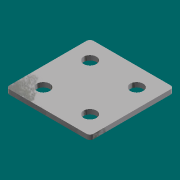
# Autodesk Inventor part: SHPTSD5-1
Saved by Autodesk Inventor 2016 (Build 200138000, 138)
## iProperties
Category: PARTsolutions
Company: MISUMI
Created: 2016-02-10
Part Number: SHPTSD5-1
Catalog Web Link: www.cadenas.de
Description: HPTSS, SHPTSS, HPTSSL, SHPTSSL, HPTSD, SHPTSD-1-Sheet Metal-1
Vendor: MISUMI
Document SubType Name: Modeling
Designer: psAdmin
Manufacturer: MISUMI
Mass: 19.1846 g
Surface Area: 28.1915 cm^2
Volume: 2.39807 cm^3
Density: 8 g/cm^3
Material: Stainless Steel
Appearance: Semi-Polished
PSOL_IDENT_0: {$CADENAS_DATA\23d-libs\misumi\metric\38_al_extrusions_blackets\hptss.prj},214 {VTYP=3D},{NB=SHPTSD5
PSOL_IDENT_1: -1},{LINA=SHPTSD5-1},{NN=HPTSS, SHPTSS, HPTSSL, SHPTSSL, HPTSD, SHPTSD-1},{DATE=17.07.2015 10:48:17}
PSOL_IDENT_2: ,{GEOMDATE=27.12.2010 00:00:00},{VERSION=},{LINEID=270},{LINESUBID=-1},{WBVAR=MAT,SHP,ALT1}  {NB=SHP
PSOL_IDENT_3: TSD5-1},{LINA=SHPTSD5-1},{KT=5},{PN=SHPTSD5-1},{TYPE=SHPTSD},{NO=5},{MAT=S},{MATALG= '','Low Carbon
PSOL_IDENT_4: Steel','S','304 Stainless Steel' },{ST=-},{SHP=SD},{ALT1=},{MASS=21},{A=36},{B=0},{T=2.0},{N=5.500},
PSOL_IDENT_5: {W=20.000},{R=1.500},{AB=SCB5-8},{NOB=4},{AN=HNTTSN5-8},{NON=4},{MASS1=11.000},{MASS2=22.000},{MASS3=
PSOL_IDENT_6: 21.000},{A1=18.000},{A2=36.000},{T1=2.300},{T2=2.000},{B1=36.000},{B2=80.000},{AB1=5-8},{AN1=5.000},
PSOL_IDENT_7: {SHPALG='SS', 'SHPTSS (Rectangular, 2 Holes)', 'SSL', 'SHPTSSL (Rectangular, 4 Holes)', 'SD'  , 'SHP
PSOL_IDENT_8: TSD (Square, 4 Holes)'},{M=5},{L=8.000},{NO1=5.000},{L1=8},{MAT1=1010 Steel (or Equivalent)},{MAT2=3
PSOL_IDENT_9: 16 Stainless Steel (or Equivalent)},{TT=1.200}
NN: HPTSS, SHPTSS, HPTSSL, SHPTSSL, HPTSD, SHPTSD-1
NT: Sheet Metal-1
NB: SHPTSD5-1
NBSYN: $PN.
LINA: SHPTSD5-1
PN: SHPTSD5-1
NO: 5
MAT: 304 Stainless Steel
ST: -
SHP: SHPTSD (Square, 4 Holes)
ALT1: w/o Fixing Bolt & Nut Set
MASS: 21
A: 36
B: 0
T: 2.0
N: 5.500
W: 20.000
R: 1.500
AB: SCB5-8
NOB: 4
AN: HNTTSN5-8
NON: 4
M: 5
L: 8.000
NO1: 5.000
L1: 8
MAT1: 1010 Steel (or Equivalent)
MAT2: 316 Stainless Steel (or Equivalent)
TT: 1.200
SUPPLIER: MISUMI
ARTICLENO: SHPTSD5-1
BOMINFO: SHPTSD5-1
CREATOR: CADENAS GmbH
Title: SHPTSD5-1
Author: Cadenas PARTsolutions
Comments: Sheet Metal-1
Autodesk Inventor part; units mm, degrees
sketch "Sketch_1" plane through (0, 0, 0) normal (0, 0, 1) x (1, 0, 0)
  arc A0 (-18, 1.5) -> (-16.5, 0) centre (-16.5, 1.5) ccw
  line L0 (-16.5, 0) -> (16.5, 0)
  arc A1 (16.5, 0) -> (18, 1.5) centre (16.5, 1.5) ccw
  line L1 (18, 1.5) -> (18, 34.5)
  arc A2 (18, 34.5) -> (16.5, 36) centre (16.5, 34.5) ccw
  line L2 (16.5, 36) -> (-16.5, 36)
  arc A3 (-16.5, 36) -> (-18, 34.5) centre (-16.5, 34.5) ccw
  line L3 (-18, 34.5) -> (-18, 1.5)
  circle A4 centre (10, 28) radius 2.75
  circle A5 centre (10, 8) radius 2.75
  circle A6 centre (-10, 28) radius 2.75
  circle A7 centre (-10, 8) radius 2.75
  constraints: 8 centre point, 8 end point, 8 point on circle
extrude "Extrusion1" add sketch "Sketch_1" against normal blind 2
ref_plane "to_bolt1_XY" through (-10, 8, 0) normal (0, 0, 1) x (1, 0, 0)
ref_plane "to_bolt1_YZ" through (-10, 8, 0) normal (1, 0, 0) x (0, 1, 0)
ref_plane "to_bolt1_ZX" through (-10, 8, 0) normal (0, 1, 0) x (0, 0, 1)
ref_plane "to_bolt2_XY" through (-10, 28, 0) normal (0, 0, 1) x (1, 0, 0)
ref_plane "to_bolt2_YZ" through (-10, 28, 0) normal (1, 0, 0) x (0, 1, 0)
ref_plane "to_bolt2_ZX" through (-10, 28, 0) normal (0, 1, 0) x (0, 0, 1)
ref_plane "to_dummy_XY" through (0, 18, 0) normal (0, 0, 1) x (1, 0, 0)
ref_plane "to_dummy_YZ" through (0, 18, 0) normal (1, 0, 0) x (0, 1, 0)
ref_plane "to_dummy_ZX" through (0, 18, 0) normal (0, 1, 0) x (0, 0, 1)
ref_plane "to_nut1_XY" through (-10, 8, -2) normal (0, 0, 1) x (1, 0, 0)
ref_plane "to_nut1_YZ" through (-10, 8, -2) normal (1, 0, 0) x (0, 1, 0)
ref_plane "to_nut1_ZX" through (-10, 8, -2) normal (0, 1, 0) x (0, 0, 1)
ref_plane "to_nut2_XY" through (-10, 28, -2) normal (0, 0, 1) x (1, 0, 0)
ref_plane "to_nut2_YZ" through (-10, 28, -2) normal (1, 0, 0) x (0, 1, 0)
ref_plane "to_nut2_ZX" through (-10, 28, -2) normal (0, 1, 0) x (0, 0, 1)
ref_plane "x1_to_bolt_XY" through (10, 8, 0) normal (0, 0, 1) x (1, 0, 0)
ref_plane "x1_to_bolt_YZ" through (10, 8, 0) normal (1, 0, 0) x (0, 1, 0)
ref_plane "x1_to_bolt_ZX" through (10, 8, 0) normal (0, 1, 0) x (0, 0, 1)
ref_plane "x2_to_bolt_XY" through (10, 28, 0) normal (0, 0, 1) x (1, 0, 0)
ref_plane "x2_to_bolt_YZ" through (10, 28, 0) normal (1, 0, 0) x (0, 1, 0)
ref_plane "x2_to_bolt_ZX" through (10, 28, 0) normal (0, 1, 0) x (0, 0, 1)
ref_plane "x3_to_bolt_XY" through (0, 10, 0) normal (0, 0, 1) x (1, 0, 0)
ref_plane "x3_to_bolt_YZ" through (0, 10, 0) normal (1, 0, 0) x (0, 1, 0)
ref_plane "x3_to_bolt_ZX" through (0, 10, 0) normal (0, 1, 0) x (0, 0, 1)
ref_plane "x4_to_bolt_XY" through (0, 30, 0) normal (0, 0, 1) x (1, 0, 0)
ref_plane "x4_to_bolt_YZ" through (0, 30, 0) normal (1, 0, 0) x (0, 1, 0)
ref_plane "x4_to_bolt_ZX" through (0, 30, 0) normal (0, 1, 0) x (0, 0, 1)
body "Solid1"
